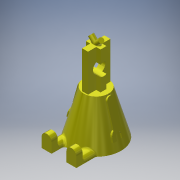
# Autodesk Inventor part: body
Saved by Autodesk Inventor 2019 (Build 230136000, 136)
## iProperties
Created: 2018-05-20
Part Number: body
Material: 一般
Document SubType Name: Modeling
Designer: uctom
Density: 1 g/cm^3
Appearance: 滑らか - 黄
Author: uctom
Autodesk Inventor part; units mm, degrees
ref_plane "YZ Plane" through (0, 0, 0) normal (1, 0, 0) x (0, 1, 0)
ref_plane "XZ Plane" through (0, 0, 0) normal (0, 1, 0) x (-1, 0, 0)
ref_plane "XY Plane" through (0, 0, 0) normal (0, 0, 1) x (1, 0, 0)
sketch "スケッチ1" plane through (0, 0, 0) normal (0, 0, 1) x (1, 0, 0)
  line L0 (0, 0) -> (0, -35)
  line L1 (0, -35) -> (-20, -35)
  line L2 (-20, -35) -> (-10, 0)
  line L3 (-10, 0) -> (0, 0)
  dimension "d1" = 35
  dimension "d2" = 20
  dimension "d3" = 10
  constraints: 8 end point, 1 parallel, 1 perpendicular, 1 vertical
  measures "d1" distance of L0.start L0.end
  measures "d2" distance of L0.end L1.end
  measures "d3" distance of L2.end L0.start
revolve "回転1" add sketch "スケッチ1" angle 360 about axis through (0, 0, 0) along (0, -1, 0)
sketch "スケッチ5" plane through (0, 0, 0) normal (0, 0, 1) x (1, 0, 0)
  line L0 (20, -35) -> (-20, -35) projected
  arc A0 (-6, -35) -> (-14, -35) centre (-10, -35) ccw
  line L1 (-14, -35) -> (-6, -35)
  line L2 (0, -35) -> (0, 0)
  dimension "d6" = 10
  dimension "d7" = 4
  constraints: 4 end point, 2 point on circle, 2 point on line, 1 centre point, 1 collinear, 1 midpoint, 1 vertical
  measures "d6" distance from line of A0.centre L2
  measures "d7" radius of A0
extrude "押し出し1" add sketch "スケッチ5" along normal blind 25
sketch "スケッチ6" plane through (0, 0, 25) normal (0, 0, 1) x (1, 0, 0)
  line L0 (-14, -35) -> (-6, -35) projected
  line L1 (-14, -27) -> (-14, -35)
  line L2 (-14, -35) -> (-6, -35)
  line L3 (-6, -35) -> (-6, -27)
  line L4 (-6, -27) -> (-14, -27)
  line L5 (-14, -27) -> (-6, -35) construction
  line L6 (-14, -35) -> (-6, -27) construction
  line L7 (-10, -45.972) -> (-10, -18.7931)
  arc A0 (-6, -27) -> (-14, -27) centre (-10, -27) ccw
  point P0 (0, 0)
  point P1 (-10, -31)
  point P2 (-10, -35)
  dimension "d8" = 8
  dimension "d9" = 8
  constraints: 14 end point, 4 midpoint, 2 parallel, 2 point on circle, 2 point on line, 2 vertical, 1 centre point, 1 collinear, 1 perpendicular, 1 other
  measures "d8" distance of L3.end L1.start
  measures "d9" distance of L2.end L3.end
extrude "足" add sketch "スケッチ6" along normal blind 5
sketch "スケッチ7" plane through (0, 0, 0) normal (0, 0, 1) x (1, 0, 0)
  line L0 (-20, -35) -> (-10, 0) projected
  point P0 (0, 0)
ref_plane "作業平面3" through (-20, -35, 0) normal (0.9615239, -0.2747211, 0) x (0.2747211, 0.9615239, 0)
sketch "スケッチ8" plane through (-20, -35, 0) normal (0.9615239, -0.2747211, 0) x (0.2747211, 0.9615239, 0)
  line L0 (0, 0) -> (36.4005, 0) projected
  line L1 (32.4005, -3) -> (12.4005, -3)
  line L2 (12.4005, -3) -> (12.4005, 3)
  line L3 (12.4005, 3) -> (32.4005, 3)
  line L4 (32.4005, 3) -> (32.4005, -3)
  line L5 (10.3271, -5.0735) -> (10.3271, 5.0735)
  arc A0 (10.3271, -5.0735) -> (10.3271, 5.0735) centre (10.3271, 0) ccw
  line L6 (10.3271, 5.0735) -> (7.3271, 5.0735)
  line L7 (7.3271, 5.0735) -> (7.3271, 2.0735)
  line L8 (7.3271, 2.0735) -> (10.3271, 2.0735)
  line L9 (10.3271, 2.0735) -> (10.3271, 5.0735)
  line L10 (10.3271, -2.0735) -> (7.3271, -2.0735)
  line L11 (7.3271, -2.0735) -> (7.3271, -5.0735)
  line L12 (7.3271, -5.0735) -> (10.3271, -5.0735)
  line L13 (10.3271, -5.0735) -> (10.3271, -2.0735)
  arc A1 (10.3271, -2.0735) -> (10.3271, 2.0735) centre (10.3271, 0) ccw
  arc A2 (32.4005, -3) -> (32.4005, 3) centre (32.4005, 0) ccw
  point P0 (39.1478, 0)
  dimension "d12" = 6
  dimension "d13" = 3
  dimension "d14" = 20
  dimension "d15" = 4
  dimension "d16" = 3
  constraints: 26 end point, 6 parallel, 6 point on circle, 3 centre point, 3 horizontal, 3 perpendicular, 2 midpoint, 1 coincident, 1 collinear, 1 point on line, 1 symmetric about line, 1 tangent, 1 vertical, 1 other
  measures "d12" distance of L3.end L1.start
  measures "d13" distance of L5.end L6.end
  measures "d14" distance of L2.end L3.end
  measures "d15" distance from line of L4 L0.end
  measures "d16" distance of L6.end L7.end
extrude "腕" add sketch "スケッチ8" along normal mid plane 5 contours L2 L3 A0 L0 | L0 A0 L1 L2 | A1 L5 A0 L3 L2 | L2 L1 A0 L5 A1 | L5 L12 L11 L10 | L8 L7 L6 L5 | A0 L3 L4 L0 | L0 L4 L1 A0 | L4 A2 L0 | L0 A2 L4
mirror "ミラー1" about plane through (0, 0, 0) normal (1, 0, 0) of "足", "押し出し1", "腕"
sketch "スケッチ9" plane through (0, 0, 0) normal (0, 1, 0) x (1, 0, 0)
  line L0 (-31.3017, 0) -> (29.5534, 0)
  line L1 (0, 27.2159) -> (0, -29.3857)
  line L2 (-5.9, 2.4) -> (5.9, 2.4)
  line L3 (5.9, 2.4) -> (5.9, -2.4)
  line L4 (5.9, -2.4) -> (-5.9, -2.4)
  line L5 (-5.9, -2.4) -> (-5.9, 2.4)
  line L6 (-2.4, 9) -> (2.4, 9)
  line L7 (2.4, 9) -> (2.4, -9)
  line L8 (2.4, -9) -> (-2.4, -9)
  line L9 (-2.4, -9) -> (-2.4, 9)
  point P0 (0, 0)
  dimension "d19" = 4.8
  dimension "d20" = 18
  dimension "d21" = 11.8
  dimension "d22" = 4.8
  constraints: 20 end point, 4 parallel, 3 horizontal, 2 perpendicular, 2 point on line, 1 vertical, 4 other
  measures "d19" distance of L6.start L6.end
  measures "d20" distance of L6.end L7.end
  measures "d21" distance of L3.end L4.end
  measures "d22" distance of L2.end L3.end
ref_plane "作業平面4" through (-15, 30, -12.5) normal (0, 1, 0) x (0, 0, 1)
extrude "押し出し4" add sketch "スケッチ9" along normal up to surface (30 mm away)
sketch "スケッチ10" plane through (5.9, 0, 2.4) normal (1, 0, 0) x (0, 0, -1)
  circle A0 centre (2.4, 15) radius 5 projected
  point P0 (2.4, 0)
extrude "押し出し5" cut sketch "スケッチ10" against normal up to surface (11.8 mm away)
sketch "スケッチ11" plane through (0, 0, 0) normal (0, 0, 1) x (1, 0, 0)
  line L0 (2.4, 30) -> (-2.4, 30) projected
  line L1 (0, 30) -> (8, 30) construction
  line L2 (0, 30) -> (1.4142, 31.4142)
  line L3 (1.4142, 31.4142) -> (-2.8284, 35.6569)
  line L4 (-2.8284, 35.6569) -> (-4.2426, 34.2426)
  line L5 (-4.2426, 34.2426) -> (0, 30)
  point P0 (0, 0)
  dimension "d34" = 6
  dimension "d35" = 45
  dimension "d38" = 2
  constraints: 10 end point, 2 parallel, 1 horizontal, 1 midpoint, 1 perpendicular
  measures "d34" distance of L3.end L2.end
  measures "d35" angle of L5 L0
  measures "d38" distance between parallel lines of L5 L3
revolve "回転2" add sketch "スケッチ11" angle 360 about axis through (-4.2426, 34.2426, 0) along (0.7071068, -0.7071068, 0)
mirror "ミラー3" about plane through (0, 0, 0) normal (1, 0, 0) of "回転2"
fillet "フィレット1" radius 2 4 edges at (10, -31, 25) (-10, -31, 25) (9.8789, -31.0018, 16.063) (-9.8789, -31.0018, 16.063)
fillet "フィレット2" radius 0.5 2 edges at (2.8284, 30, 0) (-2.8284, 30, 0)
sketch "スケッチ12" plane through (-14, -35, 30) normal (0, -1, 0) x (1, 0, 0)
  line L0 (8, -8.2853) -> (8, -7) projected
  line L1 (8, -7) -> (8, 0) projected
  line L2 (0, 0) -> (8, 0) projected
  line L3 (0, -7) -> (0, 0) projected
  line L4 (0, -14.784) -> (0, -7) projected
  arc A0 (-0.5735, -16.3028) -> (28.5735, -16.3028) centre (14, -30) ccw projected
  line L5 (28, -14.784) -> (28, -7) projected
  line L6 (28, -7) -> (28, 0) projected
  line L7 (28, 0) -> (20, 0) projected
  line L8 (20, -7) -> (20, 0) projected
  line L9 (20, -8.2853) -> (20, -7) projected
  arc A1 (17.6721, -10.34) -> (10.3279, -10.34) centre (14, -30) ccw projected
  circle A2 centre (6, -22) radius 5.1
  circle A3 centre (22, -22) radius 5.1
  circle A4 centre (6, -38) radius 5.1
  circle A5 centre (22, -38) radius 5.1
  line L10 (14, -30) -> (14, -13.3033)
  line L11 (14, -30) -> (-1.107, -30)
  dimension "d41" = 16
  dimension "d44" = 16
  dimension "d47" = 10.2
  constraints: 4 centre point, 4 end point, 2 horizontal, 2 symmetric about line, 2 vertical, 10 other
  measures "d41" distance of A2.centre A3.centre
  measures "d44" distance of A2.centre A4.centre
  measures "d47" diameter of A2
extrude "押し出し6" cut sketch "スケッチ12" against normal blind 5.5
equation "\"d22\" = d19"
